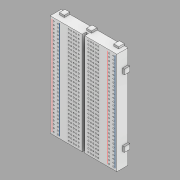
# Autodesk Inventor part: plytka_stykowa_mala
Saved by Autodesk Inventor 2021 (Build 250183000, 183)
## iProperties
Created: 2022-05-17
Part Number: plytka_stykowa_mala
Material: Generic
Document SubType Name: Modeling
Designer: agnpi
Density: 1 g/cm^3
Appearance: Smooth - White
Author: agnpi
Autodesk Inventor part; units mm, degrees
ref_plane "YZ Plane" through (0, 0, 0) normal (1, 0, 0) x (0, 1, 0)
ref_plane "XZ Plane" through (0, 0, 0) normal (0, 1, 0) x (-1, 0, 0)
ref_plane "XY Plane" through (0, 0, 0) normal (0, 0, 1) x (1, 0, 0)
sketch "Sketch1" plane through (0, 0, 0) normal (0, 0, 1) x (1, 0, 0)
  line L0 (-37.87, 0) -> (37.87, 0) projected
  line L1 (0, -57.75) -> (0, 57.75) projected
  line L2 (27.05, 41.25) -> (-27.05, 41.25)
  line L3 (-27.05, 41.25) -> (-27.05, -41.25)
  line L4 (-27.05, -41.25) -> (27.05, -41.25)
  line L5 (27.05, -41.25) -> (27.05, 41.25)
  line L6 (27.05, 41.25) -> (-27.05, -41.25) construction
  line L7 (-27.05, 41.25) -> (27.05, -41.25) construction
  point P0 (0, 0)
  dimension "d0" = 54.1
  dimension "d1" = 82.5
  constraints: 12 end point, 2 midpoint, 2 parallel, 1 horizontal, 1 perpendicular
  measures "d0" distance of L4.end L3.end
  measures "d1" distance of L3.end L2.end
extrude "Extrusion1" add sketch "Sketch1" along normal mid plane 9
sketch "Sketch2" plane through (0, 0, 4.5) normal (0, 0, 1) x (1, 0, 0)
  line L0 (-1, 41.25) -> (1, 41.25)
  line L1 (1, 41.25) -> (1, -41.25)
  line L2 (1, -41.25) -> (-1, -41.25)
  line L3 (-1, -41.25) -> (-1, 41.25)
  line L4 (27.05, -41.25) -> (27.05, 41.25) projected
  point P0 (0, 0)
  dimension "d4" = 2
  dimension "d5" = 26.05
  constraints: 8 end point, 2 parallel, 2 point on line, 1 horizontal, 1 perpendicular
  measures "d4" distance between parallel lines of L1 L3
  measures "d5" distance between parallel lines of L4 L1
extrude "Extrusion2" cut sketch "Sketch2" against normal blind 3
sketch "Sketch3" plane through (-27.05, 41.25, -4.5) normal (0, 1, 0) x (1, 0, 0)
  line L0 (3, 0) -> (7, 0)
  line L1 (7, 0) -> (7, -4.5)
  line L2 (7, -4.5) -> (3, -4.5)
  line L3 (3, -4.5) -> (3, 0)
  line L4 (47.1, 0) -> (51.1, 0)
  line L5 (51.1, 0) -> (51.1, -4.5)
  line L6 (51.1, -4.5) -> (47.1, -4.5)
  line L7 (47.1, -4.5) -> (47.1, 0)
  line L8 (25.05, 0) -> (29.05, 0)
  line L9 (29.05, 0) -> (29.05, -4.5)
  line L10 (29.05, -4.5) -> (25.05, -4.5)
  line L11 (25.05, -4.5) -> (25.05, 0)
  line L12 (54.1, 0) -> (54.1, -9) projected
  line L13 (0, 0) -> (0, -9) projected
  line L14 (28.05, -6) -> (28.05, -9) projected
  line L15 (26.05, -9) -> (26.05, -6) projected
  line L16 (0, 0) -> (54.1, 0) projected
  point P0 (27.05, -4.5)
  point P1 (27.05, 0)
  point P2 (5, 0)
  dimension "d8" = 4.5
  dimension "d9" = 4
  dimension "d10" = 4
  dimension "d11" = 4.5
  dimension "d12" = 4.5
  dimension "d13" = 4
  dimension "d14" = 3
  dimension "d15" = 3
  dimension "d17" = 1
  constraints: 24 end point, 6 parallel, 3 horizontal, 3 midpoint, 3 perpendicular, 2 point on line
  measures "d8" distance between parallel lines of L2 L0
  measures "d9" distance between parallel lines of L1 L3
  measures "d10" distance from line of L5.end L7
  measures "d11" distance between parallel lines of L6 L4
  measures "d12" distance between parallel lines of L10 L8
  measures "d13" distance from line of L9 L8.start
  measures "d14" distance between parallel lines of L12 L5
  measures "d15" distance between parallel lines of L13 L3
  measures "d17" distance between parallel lines of L15 L11
extrude "Extrusion3" add sketch "Sketch3" along normal blind 1.5
sketch "Sketch4" plane through (-27.05, -41.25, -4.5) normal (0, -1, 0) x (1, 0, 0)
  line L0 (54.1, 0) -> (0, 0) projected
  line L1 (7, 4.5) -> (7, 0) projected
  line L2 (3, 0) -> (7, 0)
  line L3 (7, 0) -> (7, 4.5)
  line L4 (7, 4.5) -> (3, 4.5)
  line L5 (3, 4.5) -> (3, 0)
  line L6 (47.1, 4.5) -> (47.1, 0) projected
  line L7 (47.1, 4.5) -> (51.1, 4.5)
  line L8 (51.1, 4.5) -> (51.1, 0)
  line L9 (51.1, 0) -> (47.1, 0)
  line L10 (47.1, 0) -> (47.1, 4.5)
  line L11 (25.05, 4.5) -> (25.05, 0) projected
  line L12 (25.05, 4.5) -> (29.05, 4.5)
  line L13 (29.05, 4.5) -> (29.05, 0)
  line L14 (29.05, 0) -> (25.05, 0)
  line L15 (25.05, 0) -> (25.05, 4.5)
  line L16 (0, 9) -> (0, 0) projected
  point P0 (27.05, 4.5)
  dimension "d20" = 4
  dimension "d21" = 4
  dimension "d22" = 4.5
  dimension "d23" = 3
  constraints: 24 end point, 6 parallel, 3 horizontal, 3 perpendicular, 2 point on line
  measures "d20" distance of L8.end L9.end
  measures "d21" distance of L13.end L14.end
  measures "d22" distance of L12.end L13.end
  measures "d23" distance between parallel lines of L16 L5
extrude "Extrusion4" cut sketch "Sketch4" against normal blind 1.5
sketch "Sketch5" plane through (27.05, -41.25, 4.5) normal (1, 0, 0) x (0, 0, -1)
  line L0 (4.5, 70.5) -> (9, 70.5)
  line L1 (9, 70.5) -> (9, 66.5)
  line L2 (9, 66.5) -> (4.5, 66.5)
  line L3 (4.5, 66.5) -> (4.5, 70.5)
  line L4 (4.5, 16) -> (9, 16)
  line L5 (9, 16) -> (9, 12)
  line L6 (9, 12) -> (4.5, 12)
  line L7 (4.5, 12) -> (4.5, 16)
  line L8 (9, 82.5) -> (0, 82.5) projected
  line L9 (9, 0) -> (0, 0) projected
  line L10 (9, 82.5) -> (9, 0) projected
  point P0 (4.5, 41.25)
  point P1 (9, 14)
  dimension "d26" = 4
  dimension "d27" = 4
  dimension "d28" = 4.5
  dimension "d29" = 12
  dimension "d30" = 12
  constraints: 16 end point, 4 parallel, 3 point on line, 2 horizontal, 2 perpendicular, 1 midpoint
  measures "d26" distance from line of L1.end L0
  measures "d27" distance of L5.end L4.end
  measures "d28" distance between parallel lines of L5 L7
  measures "d29" distance from line of L8 L0.start
  measures "d30" distance between parallel lines of L9 L6
extrude "Extrusion5" add sketch "Sketch5" along normal blind 1.5
sketch "Sketch6" plane through (-27.05, -41.25, 4.5) normal (-1, 0, 0) x (0, 0, 1)
  line L0 (-4.5, 0) -> (-4.5, 1.5) projected
  line L1 (-9, 0) -> (-9, 82.5) projected
  line L2 (-9, 70.5) -> (-4.5, 70.5) projected
  line L3 (-4.5, 70.5) -> (-9, 70.5)
  line L4 (-9, 70.5) -> (-9, 66.5)
  line L5 (-9, 66.5) -> (-4.5, 66.5)
  line L6 (-4.5, 66.5) -> (-4.5, 70.5)
  line L7 (-4.5, 16) -> (-9, 16)
  line L8 (-9, 16) -> (-9, 12)
  line L9 (-9, 12) -> (-4.5, 12)
  line L10 (-4.5, 12) -> (-4.5, 16)
  line L11 (0, 0) -> (-9, 0) projected
  point P0 (-4.5, 41.25)
  dimension "d34" = 4
  dimension "d35" = 4.5
  dimension "d36" = 4
  dimension "d37" = 12
  constraints: 16 end point, 4 parallel, 2 horizontal, 2 perpendicular, 2 point on line
  measures "d34" distance of L4.end L3.end
  measures "d35" distance between parallel lines of L1 L10
  measures "d36" distance between parallel lines of L9 L7
  measures "d37" distance between parallel lines of L11 L9
extrude "Extrusion6" cut sketch "Sketch6" against normal blind 1.5
sketch "Sketch7" plane through (0, 0, 4.5) normal (0, 0, 1) x (1, 0, 0)
  circle A0 centre (-4, 39.25) radius 0.5
  circle A1 centre (-6, 39.25) radius 0.5
  circle A2 centre (-8, 39.25) radius 0.5
  circle A3 centre (-10, 39.25) radius 0.5
  circle A4 centre (-12, 39.25) radius 0.5
  line L0 (-1, -41.25) -> (-1, 41.25) projected
  line L1 (-27.05, 41.25) -> (-27.05, -41.25) projected
  line L2 (-1, 41.25) -> (-27.05, 41.25) projected
  point P0 (0, 0)
  dimension "d40" = 1
  dimension "d41" = 1
  dimension "d42" = 1
  dimension "d43" = 1
  dimension "d44" = 1
  dimension "d45" = 3
  dimension "d46" = 2
  dimension "d47" = 2
  dimension "d48" = 2
  dimension "d49" = 2
  dimension "d50" = 15.05
  dimension "d51" = 2
  dimension "d52" = 2
  dimension "d53" = 2
  dimension "d54" = 2
  constraints: 5 centre point
  measures "d40" diameter of A0
  measures "d41" diameter of A1
  measures "d42" diameter of A2
  measures "d43" diameter of A3
  measures "d44" diameter of A4
  measures "d45" distance from line of L0 A0.centre
  measures "d46" distance of A1.centre A0.centre
  measures "d47" distance of A2.centre A1.centre
  measures "d48" distance of A3.centre A2.centre
  measures "d49" distance of A4.centre A3.centre
  measures "d50" distance from line of L1 A4.centre
  measures "d51" distance from line of L2 A4.centre
  measures "d52" distance from line of A0.centre L2
  measures "d53" distance from line of A1.centre L2
  measures "d54" distance from line of A2.centre L2
extrude "Extrusion7" cut sketch "Sketch7" against normal blind 4
pattern_linear "Rectangular Pattern1" count 30 spacing 2.7 along (0, -1, 0) of "Extrusion7"
mirror "Mirror1" about plane through (0, 0, 0) normal (1, 0, 0) of "Extrusion7", "Rectangular Pattern1"
sketch "Sketch8" plane through (0, 0, 4.5) normal (0, 0, 1) x (1, 0, 0)
  line L0 (-25.7, 39.75) -> (-25.5, 39.75)
  line L1 (-25.5, 39.75) -> (-25.5, -39.55)
  line L2 (-25.5, -39.55) -> (-25.7, -39.55)
  line L3 (-25.7, -39.55) -> (-25.7, 39.75)
  circle A0 centre (-12, -39.05) radius 0.5 projected
  circle A1 centre (-12, 39.25) radius 0.5 projected
  line L4 (-1, -41.25) -> (-1, 41.25) projected
  line L5 (-19.3, 39.75) -> (-19.5, 39.75)
  line L6 (-19.5, 39.75) -> (-19.5, -39.55)
  line L7 (-19.5, -39.55) -> (-19.3, -39.55)
  line L8 (-19.3, -39.55) -> (-19.3, 39.75)
  line L9 (0, 40.2232) -> (0, 46.1737)
  line L10 (25.7, 39.75) -> (25.5, 39.75)
  line L11 (25.5, 39.75) -> (25.5, -39.55)
  line L12 (25.5, -39.55) -> (25.7, -39.55)
  line L13 (25.7, -39.55) -> (25.7, 39.75)
  line L14 (19.3, 39.75) -> (19.5, 39.75)
  line L15 (19.3, -39.55) -> (19.3, 39.75)
  line L16 (19.5, 39.75) -> (19.5, -39.55)
  line L17 (19.5, -39.55) -> (19.3, -39.55)
  point P0 (0, 0)
  dimension "d60" = 0.2
  dimension "d61" = 0.5
  dimension "d62" = 0
  dimension "d63" = 24.5
  dimension "d65" = 90
  dimension "d66" = 90
  dimension "d67" = 90
  dimension "d68" = 90
  dimension "d69" = 19.3
  dimension "d70" = 39.75
  dimension "d71" = 39.55
  dimension "d72" = 19.5
  constraints: 34 end point, 8 symmetric about line, 2 parallel, 1 horizontal, 1 perpendicular, 1 vertical
  measures "d60" distance of L1.end L2.end
  measures "d61" vertical distance of A0.centre L1.end
  measures "d62" distance edge to line of A1 L0
  measures "d63" distance between parallel lines of L4 L1
  measures "d65" angle of L5 L4
  measures "d66" angle of L7 L4
  measures "d67" angle of L8 L5
  measures "d68" angle of L5 L6
  measures "d69" distance from line of point (0, 0) L8
  measures "d70" distance from line of point (0, 0) L5
  measures "d71" distance from line of point (0, 0) L7
  measures "d72" distance from line of point (0, 0) L6
extrude "Extrusion8" add sketch "Sketch8" along normal blind 0.02 separate body contours L0 L1 L2 L3
extrude "Extrusion9" add sketch "Sketch8" along normal blind 0.02 separate body contours L8 L7 L6 L5
extrude "Extrusion10" add sketch "Sketch8" along normal blind 0.02 separate body contours L14 L16 L17 L15
extrude "Extrusion11" add sketch "Sketch8" along normal blind 0.02 separate body contours L13 L12 L11 L10
sketch "Sketch9" plane through (0, 0, 4.5) normal (0, 0, 1) x (1, 0, 0)
  circle A0 centre (-24.25, 38.75) radius 0.5
  circle A1 centre (-20.75, 38.75) radius 0.5
  line L0 (-19.5, 39.75) -> (-19.5, -39.55) projected
  line L1 (-25.5, -39.55) -> (-25.5, 39.75) projected
  point P0 (0, 0)
  dimension "d81" = 1
  dimension "d82" = 1
  dimension "d86" = 3.5
  dimension "d87" = 1
  dimension "d88" = 1
  dimension "d89" = 1.25
  constraints: 2 centre point
  measures "d81" diameter of A0
  measures "d82" diameter of A1
  measures "d86" distance of A1.centre A0.centre
  measures "d87" vertical distance of L1.end A0.centre
  measures "d88" vertical distance of L0.start A1.centre
  measures "d89" distance from line of L0 A1.centre
extrude "Extrusion12" cut sketch "Sketch9" against normal blind 4 bodies 1
pattern_linear "Rectangular Pattern2" count 30 spacing 2.68 along (0, -1, 0) of "Extrusion12" bodies 1
mirror "Mirror3" about plane through (0, 0, 0) normal (1, 0, 0) of "Extrusion12", "Rectangular Pattern2" bodies 1
body "Solid1"
body "Solid2"
body "Solid3"
body "Solid4"
body "Solid5"
